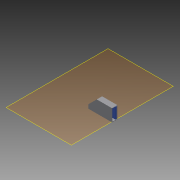
# Autodesk Inventor part: nanopc_t4_usb3
Saved by Autodesk Inventor 2013 SP2 (Build 170200200, 200)
## iProperties
Created: 2018-09-03
Part Number: nanopc_t4_usb3
Material: Generic
Document SubType Name: Modeling
Designer: alex
Density: 1 g/cm^3
Author: alex
Autodesk Inventor part; units mm, degrees
ref_plane "YZ Plane" through (0, 0, 0) normal (1, 0, 0) x (0, 1, 0)
ref_plane "XZ Plane" through (0, 0, 0) normal (0, 1, 0) x (-1, 0, 0)
ref_plane "XY Plane" through (0, 0, 0) normal (0, 0, 1) x (1, 0, 0)
ref_plane "Work Plane1" through (0, 0, 0) normal (0, 0, 1) x (1, 0, 0)
sketch "Sketch1" plane through (0, 0, 0) normal (0, 0, 1) x (1, 0, 0)
  line L0 (10.1591, -5.9453) -> (35.8591, -5.9453)
  line L1 (35.8591, -5.9453) -> (35.8591, -11.7453)
  line L2 (35.8591, -11.7453) -> (10.1591, -11.7453)
  line L3 (10.1591, -11.7453) -> (10.1591, -5.9453)
  point P0 (0, 0)
  dimension "d0" = 25.7
  dimension "d2" = 5.8
  constraints: 8 end point, 2 parallel, 1 horizontal, 1 perpendicular
  measures "d0" distance of L1.end L2.end
  measures "d2" distance of L2.end L0.start
extrude "Extrusion1" add sketch "Sketch1" along normal blind 13.2
chamfer "Chamfer1" distance 9.2 angle 45 1 edges at (10.1591, -8.8453, 13.2)
sketch "Sketch2" plane through (35.8591, -11.7453, 0) normal (1, 0, 0) x (0, 0, -1)
  line L0 (0, 5.8) -> (0, 0) projected
  line L1 (0, 5.8) -> (-13.2, 5.8) projected
  line L2 (-13.2, 0) -> (-13.2, 5.8) projected
  line L3 (0, 0) -> (-13.2, 0) projected
  line L4 (-12.8, 5.4) -> (-0.4, 5.4)
  line L5 (-0.4, 5.4) -> (-0.4, 0.4)
  line L6 (-0.4, 0.4) -> (-12.8, 0.4)
  line L7 (-12.8, 0.4) -> (-12.8, 5.4)
  point P0 (0, 11.7453)
  dimension "d8" = 0.4
  constraints: 8 end point, 3 other
  measures "d8" distance between parallel lines of L1 L4
extrude "Extrusion2" cut sketch "Sketch2" against normal blind 16 contours L4 L5 L6 L7
sketch "Sketch3" plane through (19.8591, -11.7453, 0) normal (1, 0, 0) x (0, 0, -1)
  line L0 (-12.8, 5.4) -> (-0.4, 5.4) projected
  line L1 (-12.8, 0.4) -> (-12.8, 5.4) projected
  line L2 (-0.4, 5.4) -> (-0.4, 0.4) projected
  line L3 (-12.4, 5) -> (-0.8, 5)
  line L4 (-0.8, 5) -> (-0.8, 3.6)
  line L5 (-0.8, 3.6) -> (-12.4, 3.6)
  line L6 (-12.4, 3.6) -> (-12.4, 5)
  point P0 (0, 11.7453)
  dimension "d11" = 0.4
  dimension "d12" = 0.4
  dimension "d13" = 0.4
  dimension "d14" = 1.4
  constraints: 8 end point, 2 parallel, 1 horizontal, 1 perpendicular
  measures "d11" distance between parallel lines of L1 L6
  measures "d12" distance between parallel lines of L2 L4
  measures "d13" distance between parallel lines of L0 L3
  measures "d14" distance of L5.end L3.start
extrude "Extrusion3" add sketch "Sketch3" along normal blind 16
body "Solid1"
